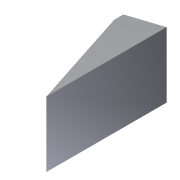
# Autodesk Inventor part: Goal Guide
Saved by Autodesk Inventor 2011 (Build 150239000, 239)
## iProperties
Created: 2014-09-14
Part Number: Goal Guide
Material: Default
Document SubType Name: Sheet Metal
Designer: Family Room
Density: 1 g/cm^3
Sheet Metal Rule: Default
Author: Family Room
Autodesk Inventor part; units mm, degrees
ref_plane "YZ Plane" through (0, 0, 0) normal (1, 0, 0) x (0, 1, 0)
ref_plane "XZ Plane" through (0, 0, 0) normal (0, 1, 0) x (-1, 0, 0)
ref_plane "XY Plane" through (0, 0, 0) normal (0, 0, 1) x (1, 0, 0)
sketch "Sketch1" plane through (0, 0, 0) normal (0, 0, 1) x (1, 0, 0)
  line L0 (6.9293, 12.8397) -> (-18.4707, 12.8397)
  line L1 (-18.4707, 12.8397) -> (-18.4707, -37.9603)
  line L2 (-18.4707, -37.9603) -> (6.9293, -37.9603)
  line L3 (6.9293, -37.9603) -> (6.9293, 12.8397)
  line L4 (-15.2957, 9.6647) -> (3.7543, 9.6647)
  line L5 (3.7543, 9.6647) -> (3.7543, -34.7853)
  line L6 (3.7543, -34.7853) -> (-15.2957, -34.7853)
  line L7 (-15.2957, -34.7853) -> (-15.2957, 9.6647)
  point P0 (0, 0)
  dimension "d0" = 25.4
  dimension "d1" = 50.8
  dimension "d2" = 3.175
  constraints: 16 end point, 4 parallel, 2 perpendicular, 1 horizontal, 3 other
  measures "d0" distance of L2.end L1.end
  measures "d1" distance of L1.end L0.end
  measures "d2" distance between parallel lines of L0 L4
extrude "Extrusion1" add sketch "Sketch1" along normal blind 254
sketch "Sketch2" plane through (-18.4707, 12.8397, 0) normal (0, 1, 0) x (1, 0, 0)
  line L0 (0, -254) -> (25.4, -254) projected
  line L1 (25.4, 0) -> (25.4, -254) projected
  line L2 (25.4, 0) -> (0, 0) projected
  line L3 (0, 0) -> (0, -254) projected
  line L4 (25.4, -254) -> (0, -175.8268)
  line L5 (25.4, -254) -> (114.3, -254) construction
  line L6 (0, -168.778) -> (25.4, -160.525)
  line L7 (25.4, -160.525) -> (25.4, -254)
  line L8 (0, -175.8268) -> (0, -168.778)
  point P0 (18.4707, 0)
  dimension "d6" = 108
  constraints: 10 end point, 3 point on line, 1 collinear, 1 horizontal, 1 perpendicular
  measures "d6" angle of L5 L4
extrude "Extrusion2" cut sketch "Sketch2" against normal blind 254 contours L3 L4 L0 | L6 L3 L2 L1
equation "\"BendRadius\" = Thickness"
equation "\"BendReliefWidth\" = Thickness"
equation "\"BendReliefDepth\" = 0.5 * Thickness"
equation "\"CornerReliefSize\" = 4 * Thickness"
equation "\"MinimumRemnant\" = 2 * Thickness"
equation "\"TransitionRadius\" = BendRadius"
equation "\"JacobiRadiusSize\" = BendRadius"
equation "\"GapSize\" = Thickness"
equation "\"Thickness\" = 3.048"
body "Solid1"
